Housing_v14 (Autodesk Fusion 360 design; units mm, degrees)
Autodesk Fusion 360 part; units mm, degrees
note: some values were not read from the file. Set by a fixed rule: the direction of a hole.
sketch "Sketch1" plane through (0, 0, 0) normal (0, 0, 1) x (1, 0, 0)
  circle A0 centre (0, 0) radius 25.4
  circle A1 centre (0, 0) radius 19.05
  circle A2 centre (0, 0) radius 22.225 construction
  line L0 (0, 0) -> (0, 25.4) construction
  point P0 (0, 22.225)
  dimension "d1" = 50.8
  dimension "d2" = 38.1
  dimension "d5" = 44.45
  constraint coincident A0.centre A1.centre
  constraint concentric A0 A2
  constraint coincident A0 L0.end
  constraint vertical L0
  constraint coincident A2 P0
  constraint coincident L0 P0
  measures "d1" diameter of A0
  measures "d2" diameter of A1
  measures "d5" diameter of A2
extrude "Extrude1" add sketch "Sketch1" along normal blind 25.4
hole "Hole1" at (0, 22.225, 0) direction (0, 0, 1) diameter 3.4163 depth 25.4 tip angle 118
thread "Thread1" "ANSI Unified Screw Threads 0.164(#8) 8-32 UNC 2B"
pattern_circular "C-Pattern1" count 3 over 360 about axis through (0, 0, 0) along (0, 0, 1) of "Hole1"
sketch "Sketch3" plane through (0, 0, 0) normal (0, 1, 0) x (1, 0, 0)
  line L0 (-25.4, -25.4) -> (25.4, -25.4)
  line L1 (-25.4, 0) -> (25.4, 0)
  line L2 (0, 0) -> (0, -12.7) construction
  line L3 (0, -12.7) -> (0, -25.4) construction
  circle A0 centre (0, -12.7) radius 3.175
  point P0 (0, -12.7)
  dimension "d12" = 6.35
  constraint coincident L2.start origin
  constraint perpendicular L1 L2
  constraint midpoint L0 L3.end
  constraint perpendicular L0 L3
  constraint coincident P0 L2.end
  constraint equal L2 L3
  measures "d12" diameter of A0
extrude "Extrude2" cut sketch "Sketch3" against normal blind 25.4
